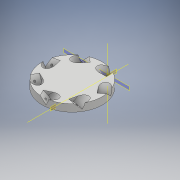
# Autodesk Inventor part: Cheek_Plate
Saved by Autodesk Inventor 2018 (Build 220112000, 112)
## iProperties
Created: 2017-08-01
Part Number: Cheek_Plate
Material: Generic
Document SubType Name: Modeling
Designer: P136265
Density: 1 g/cm^3
Appearance: Default
Author: P136265
Autodesk Inventor part; units mm, degrees
sketch "InitialGeometry" plane through (0, 0, 0) normal (0, 0, 1) x (1, 0, 0)
  circle A0 centre (0, 0) radius 100 construction
  circle A1 centre (0, 0) radius 75 construction
  circle A2 centre (0, 75) radius 25 construction
  circle A3 centre (0, 0) radius 89 construction
  line L0 (0, 75) -> (-35, 75) construction
  line L1 (0, 75) -> (35, 75) construction
  circle A4 centre (35, 75) radius 4 construction
  circle A5 centre (-35, 75) radius 4 construction
  circle A6 centre (35, 75) radius 10 construction
  circle A7 centre (-35, 75) radius 10 construction
  circle A8 centre (0, 0) radius 93
  line L2 (35, 75) -> (35, 0) construction
  dimension "d8" = 150
  dimension "d7" = 200
  dimension "d9" = 50
  dimension "d10" = 14
  dimension "d77" = 35
  dimension "d78" = 35
  dimension "d79" = 8
  dimension "d80" = 8
  dimension "d81" = 6
  dimension "d82" = 6
  dimension "d83" = 186
  dimension "d97" = 75
  constraints: 8 centre point, 6 end point, 5 coincident, 3 horizontal, 2 vertical alignment, 1 vertical, 2 other
  measures "d7" diameter of A0
  measures "d9" diameter of A2
  measures "d77" distance of L0.start L0.end
  measures "d78" distance of L0.start L1.end
  measures "d79" diameter of A4
  measures "d80" diameter of A5
  measures "d81" radial gap between concentric circles of A4 A6
  measures "d82" radial gap between concentric circles of A5 A7
  measures "d83" diameter of A8
  measures "d97" distance from line of L2.end L1
sketch "Sketch6" plane through (0, 0, 0) normal (0, 0, 1) x (1, 0, 0)
  point P0 (0, 0)
ref_plane "Work Plane3" through (0, 0, 0) normal (0, -0.7071068, 0.7071068) x (1, 0, 0)
extrude "Extrusion5" add sketch "InitialGeometry" along normal mid plane 22.5
ref_plane "Work Plane5" through (35, 0, 0) normal (1, 0, 0) x (0, 1, 0)
ref_plane "Work Plane6" through (35, 75, 0) normal (0.7071068, 0.7071068, 0) x (0, 0, -1)
ref_plane "Work Plane4" through (0, 75, 0) normal (0, 1, 0) x (-1, 0, 0)
ref_plane "CorrectPlane!!!" through (35, 0, 0) normal (0.7071068, 0, -0.7071068) x (0, 1, 0)
sketch "Sketch11" plane through (35, 0, 0) normal (0.7071068, 0, -0.7071068) x (0, 1, 0)
  ellipse E0 centre (75, 0) end of major axis (85, 0) minor radius 7.0711 construction
  circle A0 centre (75, 0) radius 3
  point P0 (0, -24.7487)
  dimension "d88" = 6
  constraints: 1 centre point, 1 coincident, 1 other
  measures "d88" diameter of A0
sketch "Sketch12" plane through (35, 0, 0) normal (0.7071068, 0, -0.7071068) x (0, 1, 0)
  arc A0 (60, 0) -> (90, 0) centre (75, 0) ccw
  line L0 (90, 0) -> (90, 30)
  line L1 (90, 30) -> (60, 30)
  line L2 (60, 30) -> (60, 0)
  point P0 (0, -24.7487)
  dimension "d92" = 30
  dimension "d94" = 30
  dimension "d95" = 30
  dimension "d96" = 30
  constraints: 6 end point, 2 point on circle, 1 centre point, 1 coincident, 1 horizontal, 1 perpendicular, 1 tangent
  measures "d92" diameter of A0
  measures "d94" distance of L0.start L0.end
  measures "d95" distance of L0.end L1.end
  measures "d96" distance of L1.end L2.end
extrude "Extrusion7" cut sketch "Sketch12" against normal blind 40
extrude "Extrusion8" cut sketch "Sketch11" along normal mid plane 50
pattern_circular "Circular Pattern1" count 7 over 360 about axis through (0, 0, 0) along (0, 0, 1) of "Extrusion7", "Extrusion8"
sketch "2d Roller Ellipse" plane through (0, 0, 0) normal (0, -0.7071068, 0.7071068) x (1, 0, 0)
  ellipse E0 centre (0, 0) end of major axis (100, 0) minor radius 70.7107 construction
  ellipse E1 centre (0, 53.033) end of major axis (25, 53.033) minor radius 17.6777 construction
  ellipse E2 centre (0, 0) end of major axis (100, 0) minor radius 70.7107 construction
  circle A0 centre (0, 45.7107) radius 22 construction
  circle A1 centre (0, 45.7107) radius 12.5 construction
  line L0 (0, 58.2107) -> (49.548, 58.2107) construction
  line L1 (49.548, 58.2107) -> (49.548, 45.7107)
  line L2 (0, 58.2107) -> (-49.548, 58.2107) construction
  line L3 (-49.548, 58.2107) -> (-49.548, 45.7107)
  line L4 (0, 45.7107) -> (-49.548, 45.7107)
  ellipse E3 centre (0, 0) end of major axis (97, 0) minor radius 67.7107 (49.548, 58.2107) -> (-49.548, 58.2107) ccw
  line L5 (0, 45.7107) -> (49.548, 45.7107)
  spline S0 degree 5 poles (125, 0) (124.9996, 8.8962) (123.6824, 17.7961) (121.0383, 26.425) (113.3824, 42.8537) (101.833, 56.8343) (95.2127, 63.1614) (80.4494, 74.6213) (63.7738, 83.0792) (54.8985, 86.6443) (36.372, 92.4116) (17.1764, 95.263) (7.3437, 95.9828) (-12.2502, 95.9826) (-31.6302, 93.1025) (-41.1422, 90.9507) (-59.3601, 85.2856) (-76.3656, 76.6479) (-84.2872, 71.6905) (-98.7984, 60.4396) (-110.4889, 46.2955) (-115.3769, 38.6773) (-122.9533, 22.3258) (-125.6666, 4.5154) (-125.6666, -4.5154) (-122.9533, -22.3258) (-115.3769, -38.6773) (-110.4889, -46.2955) (-98.7984, -60.4396) (-84.2872, -71.6905) (-76.3656, -76.6479) (-59.3601, -85.2856) (-41.1422, -90.9507) (-31.6302, -93.1025) (-12.2502, -95.9826) (7.3437, -95.9828) (17.1764, -95.263) (36.372, -92.4116) (54.8985, -86.6443) (63.7738, -83.0792) (80.4494, -74.6213) (95.2127, -63.1614) (101.833, -56.8343) (113.3824, -42.8537) (121.0383, -26.425) (123.6824, -17.7961) (124.9996, -8.8962) (125, 0) knots 0 0 0 0 0 0 0.063791 0.063791 0.063791 0.128941 0.128941 0.128941 0.197218 0.197218 0.197218 0.267663 0.267663 0.267663 0.337325 0.337325 0.337325 0.403955 0.403955 0.403955 0.468142 0.468142 0.468142 0.531858 0.531858 0.531858 0.596045 0.596045 0.596045 0.662675 0.662675 0.662675 0.732337 0.732337 0.732337 0.802782 0.802782 0.802782 0.871059 0.871059 0.871059 0.936209 0.936209 0.936209 1 1 1 1 1 1 construction
  dimension "d53" = 25
  dimension "d55" = 25
  dimension "d61" = 100
  dimension "d62" = 97
  dimension "d63" = 70.7107
  dimension "d64" = 67.7107
  dimension "d54" = 44
  dimension "d59" = 12.5
  dimension "d60" = 12.5
  constraints: 12 end point, 6 horizontal, 2 coincident, 1 centre point, 1 parallel, 1 vertical alignment, 13 other
  measures "d54" diameter of A0
  measures "d59" distance of L0.end L1.end
  measures "d60" distance of L2.end L3.end
sketch "Sketch8" plane through (49.548, 32.3223, 32.3223) normal (1, 0, 0) x (0, 0, -1)
  circle A0 centre (0, 0) radius 8
  point P0 (32.3223, -32.3223)
  dimension "d66" = 16
  constraints: 1 centre point
  measures "d66" diameter of A0
sketch "Sketch9" plane through (49.548, 32.3223, 32.3223) normal (1, 0, 0) x (0, 0, -1)
  circle A0 centre (0, 0) radius 11
  point P0 (32.3223, -32.3223)
  dimension "d71" = 22
  constraints: 1 centre point
  measures "d71" diameter of A0
sketch "Sketch10" plane through (-49.548, 32.3223, 32.3223) normal (-1, 0, 0) x (0, 0, 1)
  circle A0 centre (0, 0) radius 11
  point P0 (-32.3223, -32.3223)
  dimension "d74" = 22
  constraints: 1 centre point
  measures "d74" diameter of A0
body "Solid6"
